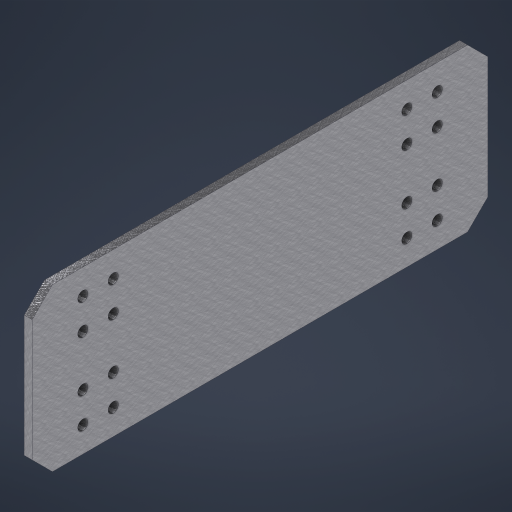
# Autodesk Inventor part: ArmBaseSupportPlates
Saved by Autodesk Inventor 2024 (Build 280153000, 153)
## iProperties
Created: 2023-10-18
Part Number: ArmBaseSupportPlates
Material: Generic
Document SubType Name: Modeling
Designer: avsar
Density: 1 g/cm^3
Appearance: Machined 02
Author: avsar
Autodesk Inventor part; units mm, degrees
ref_plane "YZ Plane" through (0, 0, 0) normal (1, 0, 0) x (0, 1, 0)
ref_plane "XZ Plane" through (0, 0, 0) normal (0, 1, 0) x (-1, 0, 0)
ref_plane "XY Plane" through (0, 0, 0) normal (0, 0, 1) x (1, 0, 0)
sketch "Sketch1" plane through (0, 0, 0) normal (1, 0, 0) x (0, 1, 0)
  line L0 (-32, 90) -> (32, 90)
  line L1 (32, 90) -> (32, -90)
  line L2 (32, -90) -> (-32, -90)
  line L3 (-32, -90) -> (-32, 90)
  line L4 (-32, 90) -> (32, -90) construction
  line L5 (32, 90) -> (-32, -90) construction
  point P0 (0, 0)
  dimension "d0" = 64
  dimension "d1" = 180
  constraints: 12 end point, 2 midpoint, 2 parallel, 1 horizontal, 1 perpendicular
  measures "d0" distance of L1.end L2.end
  measures "d1" distance of L0.end L1.end
extrude "Extrusion1" add sketch "Sketch1" along normal blind 3.175
sketch "Sketch2" plane through (3.175, 0, 0) normal (1, 0, 0) x (0, 0, -1)
  circle A0 centre (-64, -16) radius 2.5 construction
  circle A1 centre (-70, -22) radius 2
  circle A2 centre (-58, -22) radius 2
  circle A3 centre (-58, -10) radius 2
  circle A4 centre (-70, -10) radius 2
  line L0 (-90, 32) -> (-90, -32) construction
  line L1 (-90, 0) -> (90, 0) construction
  line L2 (90, -32) -> (90, 32) construction
  line L3 (90, 32) -> (-90, 32) construction
  line L4 (0, 32) -> (0, -32) construction
  line L5 (-90, -32) -> (90, -32) construction
  circle A5 centre (-64, 16) radius 2.5 construction
  circle A6 centre (-70, 22) radius 2
  circle A7 centre (-58, 22) radius 2
  circle A8 centre (-58, 10) radius 2
  circle A9 centre (-70, 10) radius 2
  circle A10 centre (64, -16) radius 2.5 construction
  circle A11 centre (70, -22) radius 2
  circle A12 centre (58, -22) radius 2
  circle A13 centre (58, -10) radius 2
  circle A14 centre (70, -10) radius 2
  circle A15 centre (64, 16) radius 2.5 construction
  circle A16 centre (70, 22) radius 2
  circle A17 centre (58, 22) radius 2
  circle A18 centre (58, 10) radius 2
  circle A19 centre (70, 10) radius 2
  point P0 (0, 0)
  dimension "d4" = 5
  dimension "d5" = 64
  dimension "d6" = 16
  dimension "d7" = 4
  dimension "d8" = 6
  dimension "d9" = 6
  dimension "d12" = 360
  constraints: 20 centre point, 15 symmetric about line, 4 end point, 4 midpoint, 24 other
  measures "d4" diameter of A0
  measures "d5" horizontal distance of point (0, 0) A0.centre
  measures "d6" vertical distance of point (0, 0) A0.centre
  measures "d7" diameter of A1
  measures "d8" horizontal distance of A0.centre A1.centre
  measures "d9" horizontal distance of A0.centre A1.centre
chamfer "Chamfer1" distance 8 angle 45 4 edges at (1.5875, 32, 90) (1.5875, -32, 90) (1.5875, -32, -90) (1.5875, 32, -90)
extrude "Extrusion2" cut sketch "Sketch2" against normal through all
body "Solid1"
